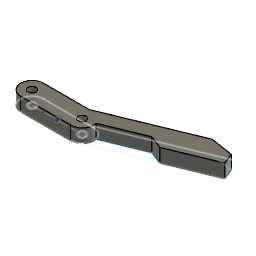
trial 2 (Autodesk Fusion 360 design; units mm, degrees)
part number: 2026-02-13-14-59-49-093
Autodesk Fusion 360 part; units mm, degrees
sketch "Sketch1" plane through (0, 0, 0) normal (0, 1, 0) x (1, 0, 0)
  line L0 (-11, -5) -> (11, -5)
  arc A0 (11, -5) -> (11, 5) centre (11, 0) ccw
  line L1 (11, 5) -> (-11, 5)
  arc A1 (-11, 5) -> (-11, -5) centre (-11, 0) ccw
  line L2 (-11, 0) -> (11, 0) construction
  circle A2 centre (-11, 0) radius 1.75
  circle A3 centre (11, 0) radius 1.75
  line L3 (9.05, 5) -> (55.3105, 23.9728)
  line L4 (55.3105, 23.9728) -> (59.2439, 14.3821)
  line L5 (59.2439, 14.3821) -> (11.9855, -5)
  line L6 (47.3582, 20.7114) -> (57.2772, 19.1775)
  line L7 (39.0063, 6.082) -> (33.2219, 8.3515)
  line L8 (33.2219, 8.3515) -> (15.8474, 1.2257)
  dimension "d1" = 22
  dimension "d2" = 5
  dimension "d3" = 3.5
  dimension "d4" = 3.5
  dimension "d5" = 157.7
  dimension "d6" = 50
  dimension "d7" = 1.95
  constraint tangent L0 A0
  constraint tangent A0 L1
  constraint parallel L0 L1
  constraint tangent L1 A1
  constraint tangent L0 A1
  constraint horizontal L2
  constraint midpoint L2 origin
  constraint concentric A1 A2
  constraint concentric A0 A3
  constraint coincident L1 L3.start
  constraint perpendicular L3 L4
  constraint coincident L0 L5.end
  constraint tangent A0 L5
  constraint perpendicular L4 L5
  constraint coincident L3 L6.start
  constraint midpoint L4 L6.end
  constraint coincident L5 L7.start
  constraint coincident A0 L8.end
  constraint parallel L5 L8
  measures "d1" distance of A1.centre A0.centre
  measures "d2" radius of A1
  measures "d3" diameter of A2
  measures "d4" diameter of A3
  measures "d5" angle of L1 L3
  measures "d6" distance of L3.start L3.end
  measures "d7" distance of A0.end L3.start
extrude "Extrude1" add sketch "Sketch1" along normal blind 3 contours L0 A0 L1 A1 | A0 L1 L3 L4 L5 L6 L7 L8
extrude "Extrude2" add 1 faces at (48.5362, 3, -13.7252) along direction (0, 1, 0) blind 3
